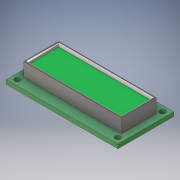
# Autodesk Inventor part: LCD
Saved by Autodesk Inventor 2019 (Build 230136000, 136)
## iProperties
Created: 2018-06-23
Part Number: LCD
Material: Generic
Document SubType Name: Modeling
Designer: Akshay
Density: 1 g/cm^3
Appearance: Default
Author: Akshay
Autodesk Inventor part; units mm, degrees
ref_plane "YZ Plane" through (0, 0, 0) normal (1, 0, 0) x (0, 1, 0)
ref_plane "XZ Plane" through (0, 0, 0) normal (0, 1, 0) x (-1, 0, 0)
ref_plane "XY Plane" through (0, 0, 0) normal (0, 0, 1) x (1, 0, 0)
sketch "Sketch1" plane through (0, 0, 0) normal (0, 1, 0) x (-1, 0, 0)
  line L0 (40, 20) -> (-40, 20)
  line L1 (-40, 20) -> (-40, -20)
  line L2 (-40, -20) -> (40, -20)
  line L3 (40, -20) -> (40, 20)
  line L4 (40, 20) -> (-40, -20) construction
  line L5 (-40, 20) -> (40, -20) construction
  point P0 (0, 0)
  dimension "d0" = 80
  dimension "d1" = 40
  constraints: 12 end point, 2 midpoint, 2 parallel, 1 horizontal, 1 perpendicular
  measures "d0" distance of L2.end L1.end
  measures "d1" distance of L1.end L0.end
extrude "Extrusion1" add sketch "Sketch1" along normal blind 3
sketch "Sketch2" plane through (0, 3, 0) normal (0, 1, 0) x (1, 0, 0)
  line L0 (-35, -12.5) -> (35, -12.5)
  line L1 (35, -12.5) -> (35, 12.5)
  line L2 (35, 12.5) -> (-35, 12.5)
  line L3 (-35, 12.5) -> (-35, -12.5)
  line L4 (-35, -12.5) -> (35, 12.5) construction
  line L5 (35, -12.5) -> (-35, 12.5) construction
  point P0 (0, 0)
  dimension "d4" = 70
  dimension "d5" = 25
  constraints: 12 end point, 2 midpoint, 2 parallel, 1 horizontal, 1 perpendicular
  measures "d4" distance of L2.end L1.end
  measures "d5" distance of L1.end L0.end
extrude "Extrusion2" add sketch "Sketch2" along normal blind 10
sketch "Sketch3" plane through (0, 13, 0) normal (0, 1, 0) x (1, 0, 0)
  line L0 (33, 10.5) -> (-33, 10.5)
  line L1 (-33, 10.5) -> (-33, -10.5)
  line L2 (-33, -10.5) -> (33, -10.5)
  line L3 (33, -10.5) -> (33, 10.5)
  line L4 (33, 10.5) -> (-33, -10.5) construction
  line L5 (-33, 10.5) -> (33, -10.5) construction
  point P0 (0, 0)
  dimension "d8" = 66
  dimension "d9" = 21
  constraints: 12 end point, 2 midpoint, 2 parallel, 1 horizontal, 1 perpendicular
  measures "d8" distance of L2.end L1.end
  measures "d9" distance of L1.end L0.end
extrude "Extrusion3" cut sketch "Sketch3" against normal blind 1.5
fillet "Fillet1" radius 1.5 4 edges at (0, 13, -10.5) (-33, 13, 0) (0, 13, 10.5) (33, 13, 0)
sketch "Sketch4" plane through (0, 3, 0) normal (0, 1, 0) x (1, 0, 0)
  line L0 (-40, 20) -> (-40, 16)
  line L1 (-40, 20) -> (-40, -20) projected
  line L2 (-40, 16) -> (-36, 16)
  circle A0 centre (-36, 16) radius 2
  line L3 (-40, 0) -> (40, 0)
  line L4 (40, -20) -> (40, 20) projected
  line L5 (40, 20) -> (-40, 20) projected
  line L6 (0, 20) -> (0, -20)
  line L7 (-40, -20) -> (40, -20) projected
  circle A1 centre (-36, -16) radius 2
  circle A2 centre (36, 16) radius 2
  circle A3 centre (36, -16) radius 2
  point P0 (0, 0)
  dimension "d13" = 4
  dimension "d14" = 4
  dimension "d15" = 4
  constraints: 8 end point, 4 centre point, 4 midpoint, 3 symmetric about line, 1 coincident, 1 perpendicular, 1 point on line, 3 other
  measures "d13" distance of L0.start L0.end
  measures "d14" distance of L0.end L2.end
  measures "d15" diameter of A0
extrude "Extrusion4" cut sketch "Sketch4" against normal blind 3 contours A0 | A1 | A2 | A3
body "Solid1"
